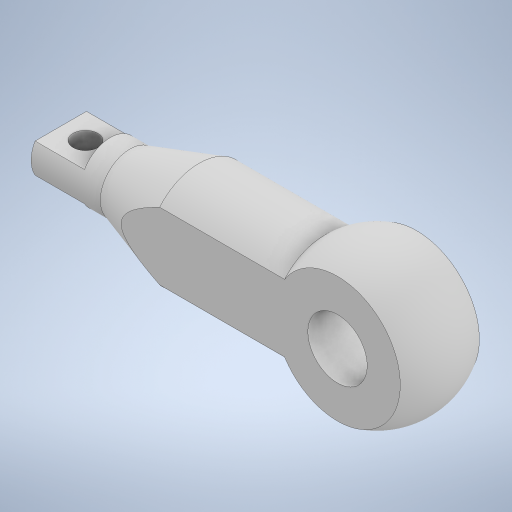
# Autodesk Inventor part: Bartosz_Zukowski_walek_04_10
Saved by Autodesk Inventor 2024 (Build 280153000, 153)
## iProperties
Created: 2024-04-10
Part Number: Bartosz_Zukowski_walek_04_10
Material: Ogólny
Document SubType Name: Modeling
Designer: student156p
Density: 1 g/cm^3
Appearance: Domyślna
Author: student156p
Autodesk Inventor part; units mm, degrees
sketch "Szkic1" plane through (0, 0, 0) normal (0, 0, 1) x (1, 0, 0)
  line L0 (0, 6) -> (14, 6)
  line L1 (14, 6) -> (14, 0)
  line L2 (14, 6) -> (28, 10.5)
  line L3 (28, 10.5) -> (28, 0)
  line L4 (28, 10.5) -> (53.2879, 10.5)
  circle A0 centre (64, 0) radius 15
  line L5 (0, 6) -> (0, 0)
  line L6 (0, 0) -> (79, 0)
  dimension "d5" = 30
  dimension "d6" = 14
  dimension "d7" = 14
  dimension "d8" = 64
  dimension "d13" = 12
  dimension "d14" = 21
  constraints: 14 end point, 2 horizontal, 2 point on circle, 1 centre point, 1 perpendicular, 1 vertical
  measures "d5" diameter of A0
  measures "d6" distance between parallel lines of L1 L5
  measures "d7" distance between parallel lines of L3 L1
  measures "d8" distance from line of A0.centre L5
  measures "d13" diameter of L0 L6
  measures "d14" diameter of L4 L6
revolve "Obrót1" add sketch "Szkic1" angle 360 about axis through (0, 0, 0) along (1, 0, 0) picked at (60.2352, 8.4613) contours L0 L1 L6 L5 | L2 L3 L6 L1 | L4 A0 L6 L3 | A0 L6
ref_plane "Płaszczyzna konstrukcyjna1" through (64, 0, -15) normal (0, 0, 1) x (1, 0, 0)
ref_plane "Płaszczyzna konstrukcyjna3" through (64, 0, 0) normal (0, 0, 1) x (1, 0, 0)
ref_plane "Płaszczyzna konstrukcyjna2" through (64, 0, 15) normal (0, 0, 1) x (1, 0, 0)
ref_plane "Płaszczyzna konstrukcyjna4" through (64, 0, 8) normal (0, 0, 1) x (1, 0, 0)
ref_plane "Płaszczyzna konstrukcyjna5" through (64, 0, -8) normal (0, 0, 1) x (1, 0, 0)
sketch "Szkic2" plane through (64, 0, -8) normal (0, 0, 1) x (1, 0, 0)
  line L0 (18, 16) -> (-68, 16)
  line L1 (-68, 16) -> (-68, -17)
  line L2 (-68, -17) -> (18, -17)
  line L3 (18, -17) -> (18, 16)
  point P0 (-64, 0)
  constraints: 8 end point, 2 parallel, 1 horizontal, 1 perpendicular
extrude "Wyciągnięcie proste1" cut sketch "Szkic2" against normal blind 10
sketch "Szkic3" plane through (64, 0, 8) normal (0, 0, 1) x (1, 0, 0)
  line L0 (20, 22) -> (-75, 22)
  line L1 (-75, 22) -> (-75, -17)
  line L2 (-75, -17) -> (20, -17)
  line L3 (20, -17) -> (20, 22)
  point P0 (-64, 0)
  constraints: 8 end point, 2 parallel, 1 horizontal, 1 perpendicular
extrude "Wyciągnięcie proste2" cut sketch "Szkic3" along normal blind 10
sketch "Szkic4" plane through (64, 0, 8) normal (0, 0, 1) x (1, 0, 0)
  arc A0 (-10.7121, -10.5) -> (-10.7121, 10.5) centre (0, 0) ccw projected
  circle A1 centre (0, 0) radius 6
  point P0 (-64, 0)
  dimension "d19" = 12
  constraints: 1 centre point, 1 coincident
  measures "d19" diameter of A1
extrude "Wyciągnięcie proste3" cut sketch "Szkic4" against normal up to surface (16 mm away)
ref_plane "Płaszczyzna konstrukcyjna6" through (7, 6, 0) normal (0, 1, 0) x (-1, 0, 0)
sketch "Szkic5" plane through (7, 6, 0) normal (0, 1, 0) x (-1, 0, 0)
  line L0 (7, 6) -> (7, -6) projected
  line L1 (7, -6) -> (-7, -6) projected
  line L2 (-7, 6) -> (-7, -6) projected
  line L3 (7, 6) -> (-7, 6) projected
  line L4 (7, -6) -> (-3, -6)
  line L5 (-3, -6) -> (-3, 6)
  line L6 (-3, 6) -> (7, 6)
  line L7 (7, 6) -> (7, -6)
  point P0 (7, 0)
  point P1 (-3, -6)
  dimension "d22" = 10
  constraints: 8 end point, 2 parallel, 1 horizontal, 1 perpendicular, 1 point on line
  measures "d22" distance between parallel lines of L0 L5
extrude "Wyciągnięcie proste4" cut sketch "Szkic5" against normal blind 3 contours L0 L1 L5 L3
ref_plane "Płaszczyzna konstrukcyjna7" through (7, 6, 0) normal (0, 1, 0) x (-1, 0, 0)
ref_plane "Płaszczyzna konstrukcyjna8" through (7, -6, 0) normal (0, 1, 0) x (-1, 0, 0)
sketch "Szkic6" plane through (7, -6, 0) normal (0, 1, 0) x (-1, 0, 0)
  point P0 (7, 0)
sketch "Szkic7" plane through (7, -6, 0) normal (0, 1, 0) x (-1, 0, 0)
  line L0 (7, 6) -> (-3, 6)
  line L1 (-3, 6) -> (-3, -6)
  line L2 (-3, -6) -> (7, -6)
  line L3 (7, -6) -> (7, 6)
  point P0 (7, 0)
  constraints: 8 end point, 2 parallel, 1 horizontal, 1 perpendicular
extrude "Wyciągnięcie proste5" cut sketch "Szkic7" along normal blind 3
sketch "Szkic8" plane through (7, 6, 0) normal (0, 1, 0) x (-1, 0, 0)
  circle A0 centre (2, 0) radius 2.5
  line L0 (7, 5.1962) -> (7, -5.1962) projected
  point P0 (7, 0)
  dimension "d28" = 5
  dimension "d29" = 5
  constraints: 1 centre point
  measures "d28" distance from line of L0 A0.centre
  measures "d29" diameter of A0
extrude "Wyciągnięcie proste6" cut sketch "Szkic8" against normal through all
